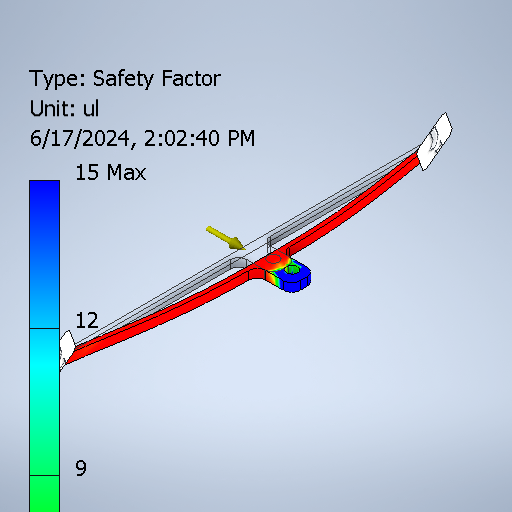
# Autodesk Inventor part: Part1
Saved by Autodesk Inventor 2025 (Build 290162010, 162A)
## iProperties
Created: 2024-06-17
Part Number: Part1
Material: ABS Plastic
Document SubType Name: Modeling
Designer: vncnt
Density: 1.06 g/cm^3
Appearance: Smooth - White
Author: vncnt
Autodesk Inventor part; units mm, degrees
ref_plane "YZ Plane" through (0, 0, 0) normal (1, 0, 0) x (0, 1, 0)
ref_plane "XZ Plane" through (0, 0, 0) normal (0, 1, 0) x (-1, 0, 0)
ref_plane "XY Plane" through (0, 0, 0) normal (0, 0, 1) x (1, 0, 0)
sketch "Sketch1" plane through (0, 0, 0) normal (0, 1, 0) x (-1, 0, 0)
  line L0 (0.5, 45) -> (-0.5, 45)
  line L1 (-0.5, 45) -> (-0.5, -45)
  line L2 (-0.5, -45) -> (0.5, -45)
  line L3 (0.5, -45) -> (0.5, 45)
  line L4 (0.5, 45) -> (-0.5, -45) construction
  line L5 (-0.5, 45) -> (0.5, -45) construction
  circle A0 centre (30.9184, 0) radius 1.905
  circle A1 centre (0, 0) radius 15
  line L6 (23.7566, 2.8287) -> (-23.7566, 2.8287)
  line L7 (-23.7566, 2.8287) -> (-23.7566, -2.8287)
  line L8 (-23.7566, -2.8287) -> (23.7566, -2.8287)
  line L9 (23.7566, -2.8287) -> (23.7566, 2.8287)
  line L10 (23.7566, 2.8287) -> (-23.7566, -2.8287) construction
  line L11 (-23.7566, 2.8287) -> (23.7566, -2.8287) construction
  line L12 (-8.7434, -12.1882) -> (-8.7434, 18.4197)
  point P0 (-0.5, 14.9917)
  point P1 (-0.5, -14.9917)
  point P2 (-14.7309, -2.8287)
  point P3 (-0.5, -2.8287)
  point P4 (-0.5, 2.8287)
  point P5 (-14.7309, 2.8287)
  point P6 (-8.7434, 2.8287)
  point P7 (-8.7434, -2.8287)
  dimension "d2" = 30
  dimension "d0" = 1
  dimension "d1" = 90
  constraints: 26 end point, 4 midpoint, 4 parallel, 2 horizontal, 2 perpendicular, 1 centre point, 1 coincident, 1 vertical, 3 other
  measures "d0" distance of L2.end L1.end
  measures "d1" distance of L1.end L0.end
extrude "Extrusion1" add sketch "Sketch1" along normal blind 2 contours L3 A1 L1 L0 | L3 L6 L1 A1 | L3 L8 L1 L6 | L1 L8 L12 L6 | L3 A1 L1 L8 | L3 L2 L1 A1
sketch "Sketch3" plane through (0, 2, 0) normal (0, 1, 0) x (1, 0, 0)
  line L0 (0.5, -45) -> (0.5, -2.8287) projected
  line L1 (0.5, 45) -> (-0.5, 45) projected
  point P0 (0, 0)
  point P1 (5.5, 0.5)
  point P2 (0.5, -14.9917)
  dimension "d5" = 5
  dimension "d13" = 44.5
  measures "d5" distance from line of L0 point (5.5, 0.5)
  measures "d13" distance from line of L1 point (5.5, 0.5)
hole "Hole1" at (5.5, 2, -0.5) direction (0, -1, 0) diameter 2.6416 depth 10.979 thread size "6-32 UNC" class "2B" standard "ANSI Unified Screw Threads"
fillet "Fillet1" radius 2 4 edges at (0.5, 1, -2.8287) (8.7434, 1, -2.8287) (8.7434, 1, 2.8287) (0.5, 1, 2.8287)
body "Solid1"
